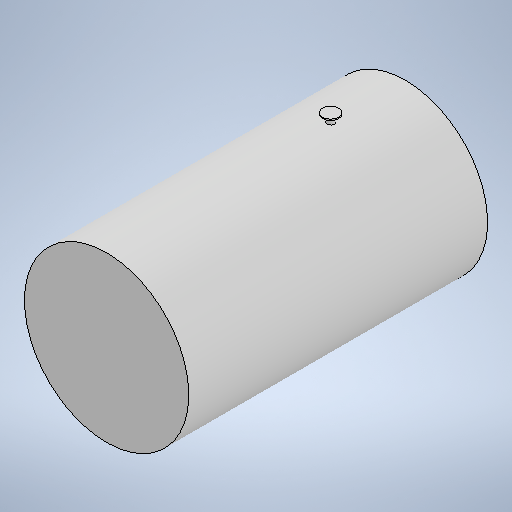
# Autodesk Inventor part: Резервуар сбора осветленной воды
Saved by Autodesk Inventor 2025 (Build 290162010, 162A)
## iProperties
Created: 2024-10-10
Part Number: Резервуар сбора осветленной воды
Material: Generic
Document SubType Name: Modeling
Designer: pokla
Density: 1 g/cm^3
Appearance: Default
Author: pokla
Autodesk Inventor part; units mm, degrees
ref_plane "XZ Plane" through (0, 0, 0) normal (0, 1, 0) x (-1, 0, 0)
sketch "Sketch1" plane through (0, 0, 0) normal (0, 1, 0) x (-1, 0, 0)
  circle A0 centre (0, 0) radius 1100
  dimension "d0" = 2200
  constraints: 1 centre point, 1 coincident
  measures "d0" diameter of A0
extrude "Extrusion1" add sketch "Sketch1" along normal blind 4000
shell "Shell1" thickness 30 removed faces 1 at (308.7984, 4000, -93.6109)
ref_plane "Work Plane1" through (0, 0, 1115) normal (0, 0, 1) x (1, 0, 0)
sketch "Sketch2" plane through (0, 0, 1115) normal (0, 0, 1) x (1, 0, 0)
  circle A0 centre (0, 3000) radius 50
  line L0 (1100, 0) -> (-1100, 0) projected
  point P0 (0, 0)
  point P1 (0, 0)
  dimension "d5" = 100
  dimension "d7" = 3000
  constraints: 1 centre point, 1 midpoint, 1 vertical alignment
  measures "d5" diameter of A0
  measures "d7" distance of point (0, 0) A0.centre
extrude "Extrusion2" add sketch "Sketch2" along normal blind 93
ref_plane "Work Plane3" through (935, 0, 0) normal (1, 0, 0) x (0, 1, 0)
sketch "Sketch5" plane through (935, 0, 0) normal (1, 0, 0) x (0, 1, 0)
  circle A0 centre (2700, 0) radius 50
  point P0 (0, 0)
  dimension "d17" = 100
  dimension "d18" = 2700
  constraints: 1 centre point, 1 horizontal alignment
  measures "d17" diameter of A0
  measures "d18" distance of point (0, 0) A0.centre
extrude "Extrusion4" add sketch "Sketch5" along normal blind 84
sketch "Sketch6" plane through (1019, 2700, 0) normal (1, 0, 0) x (0, 0, -1)
  circle A0 centre (0, 0) radius 107.5
  circle A1 centre (0, 0) radius 50 projected
  point P0 (0, -2700)
  dimension "d21" = 215
  constraints: 1 centre point, 1 coincident
  measures "d21" diameter of A0
extrude "Extrusion5" add sketch "Sketch6" along normal blind 16 contours A0 | A1
ref_plane "Work Plane4" through (0, 2600, 1028) normal (0, 0, 1) x (1, 0, 0)
sketch "Sketch8" plane through (0, 3000, 1208) normal (0, 0, 1) x (1, 0, 0)
  circle A0 centre (0, 0) radius 50 projected
  circle A1 centre (0, 0) radius 107.5
  point P0 (0, -3000)
  dimension "d27" = 215
  constraints: 1 centre point, 1 coincident
  measures "d27" diameter of A1
extrude "Extrusion7" add sketch "Sketch8" along normal blind 16 contours A0 | A1
body "Solid1"
